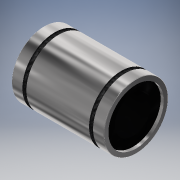
# Autodesk Inventor part: LM12UU
Saved by Autodesk Inventor 2016 (Build 200138000, 138)
## iProperties
Created: 2014-01-11
Part Number: LM12UU
Material: Generico
Document SubType Name: Modeling
Designer: Matteo
Density: 1 g/cm^3
Appearance: Steel - Polished
Author: Matteo
Autodesk Inventor part; units mm, degrees
ref_plane "YZ Plane" through (0, 0, 0) normal (1, 0, 0) x (0, 1, 0)
ref_plane "XZ Plane" through (0, 0, 0) normal (0, 1, 0) x (-1, 0, 0)
ref_plane "XY Plane" through (0, 0, 0) normal (0, 0, 1) x (1, 0, 0)
sketch "Schizzo1" plane through (0, 0, 0) normal (0, 1, 0) x (-1, 0, 0)
  line L0 (-15, 6) -> (-15, 10.5)
  line L1 (-15, 10.5) -> (-11.5, 10.5)
  line L2 (-11.5, 10.5) -> (-11.5, 10)
  line L3 (-11.5, 10) -> (-10.2, 10)
  line L4 (-10.2, 10) -> (-10.2, 10.5)
  line L5 (-10.2, 10.5) -> (0, 10.5)
  line L6 (0, 10.5) -> (0, 6)
  line L7 (0, 6) -> (-15, 6)
  line L8 (0, 0) -> (5.7518, 0)
  dimension "d0" = 12
  dimension "d2" = 21
  dimension "d3" = 15
  dimension "d4" = 11.5
  dimension "d5" = 1.3
  dimension "d6" = 20
  constraints: 18 end point, 6 parallel, 1 collinear, 1 horizontal alignment, 1 perpendicular, 1 vertical, 1 vertical alignment
  measures "d0" diameter of L7 L8
  measures "d2" diameter of L5 L8
  measures "d3" distance between parallel lines of L6 L0
  measures "d4" distance from line of L6 L1.end
  measures "d5" distance of L2.end L3.end
  measures "d6" diameter of L3 L8
revolve "Rivoluzione1" add sketch "Schizzo1" angle 360 about axis through (0, 0, 0) along (-1, 0, 0)
fillet "Raccordo1" radius 0.2 1 edges at (15, 0, -10.5)
sketch "Schizzo2" plane through (15, 0, 0) normal (1, 0, 0) x (0, 0, -1)
  circle A0 centre (0, 0) radius 10.3 projected
  circle A1 centre (0, 0) radius 9
  dimension "d13" = 18
  constraints: 1 centre point, 1 coincident
  measures "d13" diameter of A1
extrude "Estrusione2" cut sketch "Schizzo2" against normal blind 1 contours A1
mirror "Specchio1" about plane through (0, 0, 8.25) normal (-1, 0, 0)
